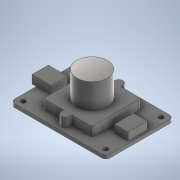
# Autodesk Inventor part: KBCR-S02MU
Saved by Autodesk Inventor 2020.4 (Build 244396000, 396)
## iProperties
Part Number: KBCR-S02MU
Material: 一般
Document SubType Name: Modeling
Designer: Masato Kubotera
Density: 2.20183 g/cm^3
Appearance: 滑らか - 黒
Mass: 10.8 g
Surface Area: 34.0637 cm^2
Volume: 4.90502 cm^3
Catalog Web Link: https://www.shikino.co.jp/products/product-kbcr-s02mu.php
Description: ReadyMade
Author: Masato Kubotera
Autodesk Inventor part; units mm, degrees
ref_plane "YZ Plane" through (0, 0, 0) normal (1, 0, 0) x (0, 1, 0)
ref_plane "XZ Plane" through (0, 0, 0) normal (0, 1, 0) x (-1, 0, 0)
ref_plane "XY Plane" through (0, 0, 0) normal (0, 0, 1) x (1, 0, 0)
sketch "スケッチ1" plane through (0, 0, 0) normal (0, 0, 1) x (1, 0, 0)
  line L0 (14, 22.5) -> (-14, 22.5)
  line L1 (-16, 20.5) -> (-16, -20.5)
  line L2 (-14, -22.5) -> (14, -22.5)
  line L3 (16, -20.5) -> (16, 20.5)
  line L4 (16, 22.5) -> (-16, -22.5) construction
  line L5 (-16, 22.5) -> (16, -22.5) construction
  line L6 (-13, 19.5) -> (13, 19.5) construction
  line L7 (13, 19.5) -> (13, -19.5) construction
  line L8 (13, -19.5) -> (-13, -19.5) construction
  line L9 (-13, -19.5) -> (-13, 19.5) construction
  line L10 (-13, 19.5) -> (13, -19.5) construction
  line L11 (13, 19.5) -> (-13, -19.5) construction
  circle A0 centre (-13, -19.5) radius 1.1
  line L12 (-16, 0) -> (16, 0) construction
  line L13 (0, 22.5) -> (0, -22.5) construction
  circle A1 centre (-13, 19.5) radius 1.1
  circle A2 centre (13, -19.5) radius 1.1
  circle A3 centre (13, 19.5) radius 1.1
  circle A4 centre (-13, -19.5) radius 2 construction
  circle A5 centre (-13, 19.5) radius 2 construction
  circle A6 centre (13, -19.5) radius 2 construction
  circle A7 centre (13, 19.5) radius 2 construction
  circle A8 centre (0, 0) radius 7.25
  arc A9 (-16, -20.5) -> (-14, -22.5) centre (-14, -20.5) ccw
  arc A10 (14, -22.5) -> (16, -20.5) centre (14, -20.5) ccw
  arc A11 (16, 20.5) -> (14, 22.5) centre (14, 20.5) ccw
  arc A12 (-14, 22.5) -> (-16, 20.5) centre (-14, 20.5) ccw
  line L14 (-10.5, 11.5) -> (10.5, 11.5)
  line L15 (11.5, 10.5) -> (11.5, -10.5)
  line L16 (10.5, -11.5) -> (-10.5, -11.5)
  line L17 (-11.5, -10.5) -> (-11.5, 10.5)
  line L18 (-11.5, 11.5) -> (11.5, -11.5) construction
  line L19 (11.5, 11.5) -> (-11.5, -11.5) construction
  line L20 (3.85, -24.5) -> (-3.85, -24.5)
  line L21 (-3.85, -24.5) -> (-3.85, -15.5)
  line L22 (-3.85, -15.5) -> (3.85, -15.5)
  line L23 (3.85, -15.5) -> (3.85, -24.5)
  line L24 (3.85, -24.5) -> (-3.85, -15.5) construction
  line L25 (-3.85, -24.5) -> (3.85, -15.5) construction
  line L26 (-4.5, 21.5) -> (4.5, 21.5)
  line L27 (4.5, 21.5) -> (4.5, 15)
  line L28 (4.5, 15) -> (-4.5, 15)
  line L29 (-4.5, 15) -> (-4.5, 21.5)
  line L30 (-4.5, 21.5) -> (4.5, 15) construction
  line L31 (4.5, 21.5) -> (-4.5, 15) construction
  arc A13 (-10.5, 11.5) -> (-11.5, 10.5) centre (-10.5, 10.5) ccw
  arc A14 (-11.5, -10.5) -> (-10.5, -11.5) centre (-10.5, -10.5) ccw
  arc A15 (10.5, -11.5) -> (11.5, -10.5) centre (10.5, -10.5) ccw
  arc A16 (11.5, 10.5) -> (10.5, 11.5) centre (10.5, 10.5) ccw
  arc A17 (-12.5, 2) -> (-12.5, -2) centre (-12.5, 0) ccw
  line L32 (-12.5, 2) -> (-11.5, 2)
  line L33 (-12.5, -2) -> (-11.5, -2)
  arc A18 (12.5, -2) -> (12.5, 2) centre (12.5, 0) ccw
  line L34 (12.5, 2) -> (11.5, 2)
  line L35 (12.5, -2) -> (11.5, -2)
  point P0 (0, -20)
  point P1 (0, 18.25)
  point P2 (3.85, -22.5)
  point P3 (-3.85, -22.5)
  dimension "d0" = 32
  dimension "d1" = 45
  dimension "d5" = 2.2
  dimension "d6" = 4
  dimension "d34" = 2
  dimension "d40" = 26
  dimension "d41" = 39
  dimension "d42" = 14.5
  dimension "d43" = 23
  dimension "d44" = 23
  dimension "d45" = 7.7
  dimension "d46" = 9
  dimension "d47" = 2
  dimension "d48" = 9
  dimension "d49" = 6.5
  dimension "d50" = 1
  dimension "d57" = 1
  dimension "d58" = 2
  dimension "d59" = 1
  constraints: 72 end point, 21 point on line, 20 point on circle, 19 centre point, 17 tangent, 14 midpoint, 11 symmetric about line, 10 parallel, 7 perpendicular, 6 equal radius, 5 horizontal, 3 coincident, 8 other
  measures "d0" distance of L5.end L4.end
  measures "d1" distance of L4.end L5.start
  measures "d5" diameter of A0
  measures "d6" diameter of A4
  measures "d34" radius of A9
  measures "d40" distance of L7.end L8.end
  measures "d41" distance of L8.end L6.start
  measures "d42" diameter of A8
  measures "d43" distance of L18.end L19.end
  measures "d44" distance of L19.start L18.end
  measures "d45" distance of L21.end L22.end
  measures "d46" distance of L22.end L20.start
  measures "d47" distance between parallel lines of L20 L2
  measures "d48" distance of L27.end L28.end
  measures "d49" distance of L26.end L27.end
  measures "d50" distance between parallel lines of L26 L0
  measures "d57" radius of A13
  measures "d58" radius of A17
  measures "d59" distance of L32.start L32.end
extrude "押し出し1" add sketch "スケッチ1" along normal blind 1.6 contours A11 L3 A10 L2 L23 L22 L21 A9 L1 A12 L0 | L2 L21 L22 L23 | A8 | L14 A16 L15 A15 L16 A14 L17 A13 | L17 L33 A17 L32 | L34 A18 L35 L15 | L26 L27 L28 L29
extrude "押し出し2" add sketch "スケッチ1" along normal blind 6.1 contours L14 A16 L15 A15 L16 A14 L17 A13 | L17 L33 A17 L32 | L34 A18 L35 L15
extrude "押し出し3" add sketch "スケッチ1" along normal blind 18 contours A8
extrude "押し出し4" add sketch "スケッチ1" along normal blind 5.5 contours L23 L20 L21 L2 | L2 L21 L22 L23
extrude "押し出し5" cut sketch "スケッチ1" along normal blind 1.6 contours L23 L20 L21 L2
extrude "押し出し6" add sketch "スケッチ1" along normal blind 5.3 contours L26 L27 L28 L29
